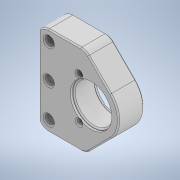
# Autodesk Inventor part: BearingStandoff2_2
Saved by Autodesk Inventor 2020 (Build 240168000, 168)
## iProperties
Created: 2020-02-02
Part Number: BearingStandoff2_2
Material: Generic
Document SubType Name: Modeling
Designer: srini
Density: 1 g/cm^3
Appearance: Default
Author: srini
Autodesk Inventor part; units mm, degrees
ref_plane "YZ Plane" through (0, 0, 0) normal (1, 0, 0) x (0, 1, 0)
ref_plane "XZ Plane" through (0, 0, 0) normal (0, 1, 0) x (-1, 0, 0)
ref_plane "XY Plane" through (0, 0, 0) normal (0, 0, 1) x (1, 0, 0)
sketch "Sketch1" plane through (0, 0, 0) normal (0, 0, 1) x (1, 0, 0)
  circle A0 centre (0, 0) radius 14.3002
  circle A1 centre (-31.75, 25.4) radius 3.3734
  line L0 (-31.75, 25.4) -> (-31.75, 19.7374)
  line L1 (-39.8734, 33.5234) -> (20.6502, 33.5234)
  line L2 (20.6502, 33.5234) -> (20.6502, -33.5234)
  line L3 (20.6502, -33.5234) -> (-39.8734, -33.5234)
  line L4 (-39.8734, -33.5234) -> (-39.8734, 33.5234)
  circle A2 centre (-31.75, 0) radius 3.3734
  line L5 (-31.75, 0) -> (-31.75, -5.6626)
  circle A3 centre (-31.75, -25.4) radius 3.3734
  line L6 (-31.75, -25.4) -> (-31.75, -31.0626)
  circle A4 centre (0, 0) radius 20.6502
  line L7 (-4.3196, 33.5234) -> (14.6019, 14.6019)
  line L8 (-4.3196, -33.5234) -> (14.6019, -14.6019)
  line L9 (-20.6502, 14.3879) -> (-20.6502, -18.7109) construction
  circle A5 centre (0, 0) radius 15.5575 construction
  line L10 (-15.5575, 17.5538) -> (-15.5575, -20.664) construction
  line L11 (-39.8734, 26.8016) -> (-41.275, 25.4)
  line L12 (-41.275, 25.4) -> (-41.275, -25.4)
  line L13 (-41.275, -25.4) -> (-39.8734, -26.8016)
  line L14 (-39.8734, -26.8016) -> (-39.8734, 26.8016)
  dimension "d0" = 28.6004
  dimension "d1" = 25.4
  dimension "d2" = 6.7469
  dimension "d6" = 25.4
  dimension "d11" = 8.1234
  dimension "d12" = 8.1234
  dimension "d13" = 8.1234
  dimension "d14" = 20.6502
  dimension "d15" = 45
  dimension "d16" = 45
  dimension "d43" = 31.115
  dimension "d45" = 31.75
  dimension "d46" = 16.1925
  dimension "d47" = 50.8
  dimension "d48" = 25.4
  dimension "d49" = 135
  dimension "d50" = 9.525
  constraints: 30 end point, 6 centre point, 5 tangent, 5 vertical, 3 coincident, 2 parallel, 2 perpendicular, 2 point on circle, 2 point on line, 1 collinear, 1 horizontal, 8 other
  measures "d0" diameter of A0
  measures "d1" vertical distance of L0.start point (0, 0)
  measures "d2" diameter of A1
  measures "d6" distance of L0.start L5.start
  measures "d11" distance from line of L0.start L1
  measures "d12" distance from line of L3 L6.start
  measures "d13" distance from line of L4 L0.start
  measures "d14" distance from line of L2 A0.centre
  measures "d15" angle of L7 L1
  measures "d16" angle of L3 L8
  measures "d43" diameter of A5
  measures "d45" horizontal distance of point (0, 0) L0.start
  measures "d46" distance from line of L5.start L10
  measures "d47" distance of L11.end L12.end
  measures "d48" vertical distance of L11.end point (0, 0)
  measures "d49" angle of L12 L11
  measures "d50" distance from line of L12 L5.start
extrude "Extrusion1" add sketch "Sketch1" along normal blind 19.05 contours L1 L7 A4 L8 L3 L4 | L4 L13 L12 L11 | A4
fillet "Fillet1" radius 8.1234 4 edges at (-39.8734, -33.5234, 9.525) (-4.3196, -33.5234, 9.525) (-39.8734, 33.5234, 9.525) (-4.3196, 33.5234, 9.525)
sketch "Sketch2" plane through (0, 0, 19.05) normal (0, 0, 1) x (1, 0, 0)
  circle A0 centre (-9.0233, 15.6289) radius 2.0193
  line L0 (0, 0) -> (6.2322, 0)
  circle A1 centre (-9.0234, -15.6289) radius 2.0193
  circle A2 centre (18.0467, 0) radius 2.0193
  dimension "d20" = 18.0467
  dimension "d21" = 4.0386
  dimension "d22" = 120
  dimension "d25" = 360
  constraints: 3 centre point, 2 end point, 1 horizontal, 7 other
  measures "d20" distance of L0.start A0.centre
  measures "d21" diameter of A0
extrude "Extrusion2" cut sketch "Sketch2" against normal through all contours A0 | A1
sketch "Sketch3" plane through (0, 0, 19.05) normal (0, 0, 1) x (1, 0, 0)
  circle A0 centre (0, 0) radius 15.5702
  dimension "d29" = 31.1404
  constraints: 1 centre point, 1 coincident
  measures "d29" diameter of A0
extrude "Extrusion3" cut sketch "Sketch3" against normal blind 1.6256
sketch "Sketch4" plane through (0, 0, 0) normal (0, 0, -1) x (-1, 0, 0)
  circle A0 centre (0, 0) radius 15.5702
  dimension "d32" = 31.1404
  constraints: 1 centre point, 1 coincident
  measures "d32" diameter of A0
extrude "Extrusion4" cut sketch "Sketch4" against normal blind 1.6256
chamfer "Chamfer1" distance 0.889 angle 45 30 edges at (-19.7782, 33.5234, 19.05) (-37.097, 31.62, 19.05) (-37.097, -31.62, 19.05) (-19.7782, -33.5234, 19.05) (-4.5758, -32.9051, 19.05) (6.3308, -22.873, 19.05) (20.6502, 0, 19.05) (6.3308, 22.873, 19.05) (-4.5758, 32.9051, 19.05) (-35.1234, 25.4, 19.05) (-35.1234, 0, 19.05) (-35.1234, -25.4, 19.05) (-11.0426, 15.6289, 19.05) (-11.0427, -15.6289, 19.05) (-14.3002, 0, 17.4244) (-14.3002, 0, 1.6256) (-11.0426, 15.6289, 0) (-11.0427, -15.6289, 0) (-35.1234, 25.4, 0) (-35.1234, 0, 0) (-35.1234, -25.4, 0) (-19.7782, 33.5234, 0) (-37.097, 31.62, 0) (-37.097, -31.62, 0) (-19.7782, -33.5234, 0) (-4.5758, -32.9051, 0) (6.3308, -22.873, 0) (20.6502, 0, 0) (6.3308, 22.873, 0) (-4.5758, 32.9051, 0)
chamfer "Chamfer2" distance 3.175 angle 45 2 edges at (-41.275, 0, 19.05) (-41.275, 0, 0)
equation "\"d12\" = d11"
equation "\"d13\" = d11"
equation "\"d48\" = 0.5 * d47"
equation "\"d19\" = d11"
body "Solid1"
